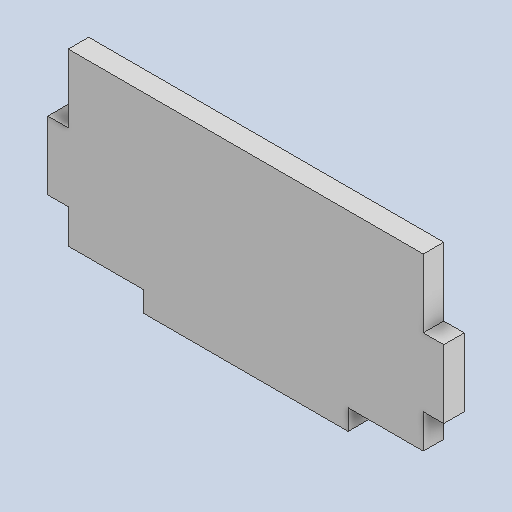
# Autodesk Inventor part: bottom_hinge_002
Saved by Autodesk Inventor 2025.2 (Build 292293000, 293)
## iProperties
Created: 2025-03-24
Part Number: bottom_hinge_002
Material: Generic
Document SubType Name: Sheet Metal
Designer: Caspe
Density: 1 g/cm^3
Sheet Metal Rule: Default_mm
Appearance: Default
Flat Pattern Width: 2.8 cm
Flat Pattern Length: 5.8 cm
Flat Pattern Area: 16.24 cm^2
Sheet Metal Width: 28,000 mm
Sheet Metal Length: 58,000 mm
Sheet Metal Area: 1624,000 mm^2
Author: Caspe
Autodesk Inventor part; units mm, degrees
ref_plane "YZ Plane" through (0, 0, 0) normal (1, 0, 0) x (0, 1, 0)
ref_plane "XZ Plane" through (0, 0, 0) normal (0, 1, 0) x (-1, 0, 0)
ref_plane "XY Plane" through (0, 0, 0) normal (0, 0, 1) x (1, 0, 0)
sketch "Sketch1" plane through (0, 0, 0) normal (0, 0, 1) x (1, 0, 0)
  line L0 (0, 0) -> (52, 0)
  line L1 (52, 0) -> (52, 25)
  line L2 (52, 25) -> (0, 25)
  line L3 (0, 25) -> (0, 0)
  line L4 (11, 0) -> (41, 0)
  line L5 (41, 0) -> (41, -3)
  line L6 (41, -3) -> (11, -3)
  line L7 (11, -3) -> (11, 0)
  line L8 (0, 5) -> (-3, 5)
  line L9 (-3, 5) -> (-3, 15)
  line L10 (-3, 15) -> (0, 15)
  line L11 (0, 15) -> (0, 5)
  line L12 (26, 25) -> (26, 0)
  line L13 (52, 5) -> (55, 5)
  line L14 (55, 5) -> (55, 15)
  line L15 (55, 15) -> (52, 15)
  point P0 (0, 15)
  point P1 (41, 0)
  point P2 (52, 5)
  point P3 (0, 15)
  dimension "d0" = 52
  dimension "d1" = 30
  dimension "d2" = 3
  dimension "d3" = 25
  dimension "d4" = 3
  dimension "d5" = 10
  dimension "d6" = 5
  measures "d0" distance of L2.end L1.end
  measures "d1" distance of L5.end L6.end
  measures "d2" distance of L4.end L5.end
  measures "d3" distance between parallel lines of L2 L0
  measures "d4" distance of L9.end L10.end
  measures "d5" distance of L8.end L9.end
  measures "d6" distance between parallel lines of L0 L8
extrude "Plate1" add sketch "Sketch1" along normal blind 3
equation "\"d0\" = A_width + 2 * A_joint_tolerance"
equation "\"d2\" = plate_thickness"
equation "\"d4\" = plate_thickness"
equation "\"d7\" = Thickness"
equation "\"Thickness\" = plate_thickness"
equation "\"BendRadius\" = Thickness"
equation "\"BendReliefWidth\" = Thickness"
equation "\"BendReliefDepth\" = 0.5 * Thickness"
equation "\"CornerReliefSize\" = 4 * Thickness"
equation "\"MinimumRemnant\" = 2 * Thickness"
equation "\"TransitionRadius\" = BendRadius"
equation "\"JacobiRadiusSize\" = BendRadius"
equation "\"GapSize\" = Thickness"
equation "\"A_width\" = 46"
equation "\"A_joint_diameter\" = 16"
equation "\"l___________\" = 0"
equation "\"l__________\" = 0"
equation "\"l_________\" = 0"
equation "\"rivet_diameter\" = 3.35"
equation "\"plate_thickness\" = 3"
equation "\"l________\" = 0"
equation "\"A_joint_tolerance\" = 3"
equation "\"A_B_spacing\" = 2"
equation "\"L_Piston_Bottom\" = 21"
equation "\"L_Piston_Top\" = 25"
equation "\"thin_plate\" = 1.5"
body "Solid1"
